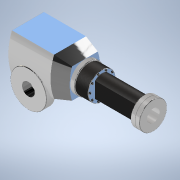
# Autodesk Inventor part: Part4
Saved by Autodesk Inventor 2022 (Build 260153000, 153)
## iProperties
Created: 2023-11-30
Part Number: Part4
Material: Generic
Document SubType Name: Modeling
Designer: harshidd
Density: 1 g/cm^3
Appearance: Aluminum - Polished
Author: harshidd
Autodesk Inventor part; units mm, degrees
sketch "Sketch1" plane through (0, 0, 0) normal (0, 0, 1) x (1, 0, 0)
  line L0 (0, 0) -> (0, 45) construction
  line L1 (0, 0) -> (0, -45) construction
  line L2 (0, 45) -> (37.5, 45)
  line L3 (37.5, 45) -> (-37.5, 45)
  line L4 (37.5, -45) -> (-37.5, -45)
  arc A0 (-37.5, 45) -> (-37.5, -45) centre (79.119038, 0) ccw
  arc A1 (37.5, -45) -> (37.5, 45) centre (-79.119038, 0) ccw
  dimension "d0" = 45
  dimension "d1" = 37.5
  dimension "d2" = 75
  dimension "d3" = 75
  dimension "d4" = 125
  dimension "d5" = 125
  constraints: 10 end point, 4 point on circle, 2 centre point, 2 vertical, 1 collinear, 1 horizontal, 1 point on line
  measures "d0" distance of L0.start L0.end
  measures "d1" distance of L0.end L2.end
  measures "d2" distance of L2.end L3.end
  measures "d3" distance of L4.start L4.end
  measures "d4" radius of A0
  measures "d5" radius of A1
sketch "Sketch1 outline for Extrusion1" plane through (0, 0, 0) normal (0, 0, 1) x (1, 0, 0)
  arc A0 (37.5, -45) -> (37.5, 45) centre (-79.119038, 0) ccw
  line L0 (-37.5, -45) -> (37.5, -45)
  arc A1 (-37.5, 45) -> (-37.5, -45) centre (79.119038, 0) ccw
  line L1 (37.5, 45) -> (-37.5, 45)
extrude "Extrusion1" add sketch "Sketch1 outline for Extrusion1" along normal blind 100
ref_plane "Work Plane1" through (0, 0, 135) normal (0, 0, 1) x (1, 0, 0)
sketch "Sketch2" plane through (0, 0, 135) normal (0, 0, 1) x (1, 0, 0)
  line L0 (37.5, 45) -> (-37.5, 45)
  arc A0 (-37.5, 45) -> (-37.5, -45) centre (79.119038, 0) ccw
  line L1 (-37.5, -45) -> (37.5, -45)
  arc A1 (37.5, -45) -> (37.5, 45) centre (-79.119038, 0) ccw
  line L2 (-30.425474, 35) -> (30.425474, 35)
  arc A2 (30.425474, -35) -> (30.425474, 35) centre (-79.119038, 0) ccw
  line L3 (30.425474, -35) -> (-30.425474, -35)
  arc A3 (-30.425474, 35) -> (-30.425474, -35) centre (79.119038, 0) ccw
  point P0 (0, 0)
  dimension "d9" = 10
  constraints: 4 end point, 4 point on circle, 2 centre point, 3 other
  measures "d9" distance between parallel lines of L0 L2
sketch "Sketch2 outline for Loft1" plane through (0, 0, 135) normal (0, 0, 1) x (1, 0, 0)
  line L0 (-30.425474, 35) -> (30.425474, 35)
  arc A0 (30.425474, 35) -> (30.425474, -35) centre (-79.119038, 0) cw
  line L1 (30.425474, -35) -> (-30.425474, -35)
  arc A1 (-30.425474, -35) -> (-30.425474, 35) centre (79.119038, 0) cw
loft "Loft1" add profiles "Sketch2 outline for Loft1" section 1 edges at (0, 45, 100) (-45.880962, 0, 100) (0, -45, 100) (45.880962, 0, 100)
sketch "Sketch3" plane through (-30.425474, 35, 135) normal (0, 0, 1) x (1, 0, 0)
  circle A0 centre (30.425474, -35) radius 34.5
  dimension "d14" = 69
  constraints: 1 centre point, 1 coincident
  measures "d14" diameter of A0
sketch "Sketch3 outline for Extrusion2" plane through (-30.425474, 35, 135) normal (0, 0, 1) x (1, 0, 0)
  circle A0 centre (30.425474, -35) radius 34.5
extrude "Extrusion2" add sketch "Sketch3 outline for Extrusion2" along normal blind 10
sketch "Sketch4" plane through (0, 0, 145) normal (0, 0, 1) x (1, 0, 0)
  circle A0 centre (0, 0) radius 34.5 projected
  circle A1 centre (0, 0) radius 32.5
  dimension "d17" = 2
  constraints: 1 centre point
  measures "d17" radial gap between concentric circles of A0 A1
sketch "Sketch4 outline for Extrusion3" plane through (0, 0, 145) normal (0, 0, 1) x (1, 0, 0)
  circle A0 centre (0, 0) radius 32.5
extrude "Extrusion3" add sketch "Sketch4 outline for Extrusion3" along normal blind 30
sketch "Sketch5" plane through (0, 0, 175) normal (0, 0, 1) x (1, 0, 0)
  line L0 (0, 0) -> (29, 0) construction
  circle A0 centre (29, 0) radius 2.5
  circle A1 centre (29, 0) radius 1.5
  dimension "d20" = 29
  dimension "d21" = 5
  dimension "d22" = 1
  constraints: 2 centre point, 2 end point, 1 coincident, 1 horizontal
  measures "d20" distance of L0.start L0.end
  measures "d21" diameter of A0
  measures "d22" radial gap between concentric circles of A0 A1
sketch "Sketch5 outline for Extrusion4" plane through (0, 0, 175) normal (0, 0, 1) x (1, 0, 0)
  circle A0 centre (29, 0) radius 2.5
  circle A1 centre (29, 0) radius 1.5
extrude "Extrusion4" add sketch "Sketch5 outline for Extrusion4" along normal blind 2
pattern_circular "Circular Pattern1" count 10 over 360 about axis through (0, 0, 145) along (0, 0, 1) of "Extrusion4"
sketch "Sketch6" plane through (0, 0, 175) normal (0, 0, 1) x (1, 0, 0)
  line L0 (0, 0) -> (16, 0) construction
  line L1 (16, 0) -> (16, 18.5) construction
  line L2 (16, 18.5) -> (16, -18.5)
  line L3 (0, 0) -> (0, -6.981731) construction
  line L4 (-16, 18.5) -> (-16, -18.5)
  arc A0 (16, 18.5) -> (-16, 18.5) centre (0, 4.898529) ccw
  arc A1 (-16, -18.5) -> (16, -18.5) centre (0, -4.898529) ccw
  dimension "d28" = 16
  dimension "d29" = 18.5
  dimension "d30" = 37
  dimension "d31" = 21
  dimension "d32" = 21
  constraints: 10 end point, 4 point on circle, 2 centre point, 2 symmetric about line, 2 vertical, 1 horizontal, 1 point on line
  measures "d28" distance of L0.start L0.end
  measures "d29" distance of L0.end L1.end
  measures "d30" distance of L1.end L2.end
  measures "d31" radius of A0
  measures "d32" radius of A1
sketch "Sketch6 outline for Extrusion5" plane through (0, 0, 175) normal (0, 0, 1) x (1, 0, 0)
  line L0 (16, 18.5) -> (16, -18.5)
  arc A0 (16, -18.5) -> (-16, -18.5) centre (0, -4.898529) cw
  line L1 (-16, -18.5) -> (-16, 18.5)
  arc A1 (-16, 18.5) -> (16, 18.5) centre (0, 4.898529) cw
extrude "Extrusion5" add sketch "Sketch6 outline for Extrusion5" along normal blind 100
sketch "Sketch7" plane through (0, 0, 275) normal (0, 0, 1) x (1, 0, 0)
  circle A0 centre (0, 0) radius 32.5 projected
sketch "Sketch7 outline for Extrusion6" plane through (0, 0, 275) normal (0, 0, 1) x (1, 0, 0)
  circle A0 centre (0, 0) radius 32.5
extrude "Extrusion6" add sketch "Sketch7 outline for Extrusion6" along normal blind 10
sketch "Sketch8" plane through (0, 0, 285) normal (0, 0, 1) x (1, 0, 0)
  circle A0 centre (0, 0) radius 32.5 projected
  circle A1 centre (0, 0) radius 31.5
  dimension "d37" = 1
  constraints: 1 centre point
  measures "d37" radial gap between concentric circles of A0 A1
sketch "Sketch8 outline for Extrusion7" plane through (0, 0, 285) normal (0, 0, 1) x (1, 0, 0)
  circle A0 centre (0, 0) radius 31.5
extrude "Extrusion7" add sketch "Sketch8 outline for Extrusion7" along normal blind 1
sketch "Sketch9" plane through (0, 0, 286) normal (0, 0, 1) x (1, 0, 0)
  circle A0 centre (0, 0) radius 32.5 projected
sketch "Sketch9 outline for Extrusion8" plane through (0, 0, 286) normal (0, 0, 1) x (1, 0, 0)
  circle A0 centre (0, 0) radius 32.5
extrude "Extrusion8" add sketch "Sketch9 outline for Extrusion8" along normal blind 10
ref_plane "Work Plane2" through (-37.5, -45, 50) normal (1, 0, 0) x (0, 1, 0)
sketch "Sketch10" plane through (-37.5, -45, 50) normal (1, 0, 0) x (0, 1, 0)
  line L0 (0, -50) -> (0, 50) projected
  circle A0 centre (0, 0) radius 42.5
  point P0 (45, -50)
  dimension "d42" = 85
  constraints: 1 centre point, 1 midpoint
  measures "d42" diameter of A0
sketch "Sketch10 outline for Extrusion9" plane through (-37.5, -45, 50) normal (1, 0, 0) x (0, 1, 0)
  circle A0 centre (0, 0) radius 42.5
extrude "Extrusion9" add sketch "Sketch10 outline for Extrusion9" along normal mid plane 21
sketch "Sketch11" plane through (-27, -45, 50) normal (1, 0, 0) x (0, 0, -1)
  line L0 (50, 0) -> (-50, 0) construction
  line L1 (0, 0) -> (0, -30) construction
  line L2 (20, 0) -> (20, -30)
  line L3 (-20, 0) -> (-20, -30)
  arc A0 (-20, -30) -> (20, -30) centre (0, -7.63932) ccw
  line L4 (-20, 0) -> (20, 0)
  point P0 (50, 45)
  dimension "d45" = 30
  dimension "d46" = 20
  dimension "d47" = 30
  constraints: 8 end point, 2 point on circle, 2 symmetric about line, 1 centre point, 1 collinear, 1 midpoint, 1 parallel, 1 vertical
  measures "d45" distance of L1.start L1.end
  measures "d46" distance between parallel lines of L1 L2
  measures "d47" radius of A0
sketch "Sketch11 outline for Extrusion10" plane through (-27, -45, 50) normal (1, 0, 0) x (0, 0, -1)
  line L0 (20, 0) -> (20, -30)
  arc A0 (20, -30) -> (-20, -30) centre (0, -7.63932) cw
  line L1 (-20, -30) -> (-20, 0)
  line L2 (-20, 0) -> (20, 0)
extrude "Extrusion10" add sketch "Sketch11 outline for Extrusion10" along normal blind 35
ref_plane "Work Plane3" through (8, -45, 50) normal (0, 0, 1) x (1, 0, 0)
sketch "Sketch12" plane through (8, -45, 50) normal (0, 0, 1) x (1, 0, 0)
  line L0 (0, -30) -> (0, 0)
  line L1 (0, 0) -> (0, -42)
  line L2 (0, 0) -> (25, 0)
  line L3 (-45.5, 0) -> (29.5, 0)
  arc A0 (0, -42) -> (25, 0) centre (-29.839254, 4.201937) ccw
  point P0 (-8, 45)
  dimension "d50" = 42
  dimension "d51" = 25
  dimension "d52" = 55
  constraints: 4 end point, 2 point on circle, 1 centre point, 1 collinear, 1 point on line
  measures "d50" distance of L0.end L1.end
  measures "d51" distance of L0.end L2.end
  measures "d52" radius of A0
sketch "Sketch12 outline for Extrusion11" plane through (8, -45, 50) normal (0, 0, 1) x (1, 0, 0)
  line L0 (25, 0) -> (0, 0)
  arc A0 (0, -42) -> (25, 0) centre (-29.839254, 4.201937) ccw
  line L1 (0, 0) -> (0, -42)
extrude "Extrusion11" add sketch "Sketch12 outline for Extrusion11" along normal mid plane 40
sketch "Sketch13" plane through (8, -87, 30) normal (-1, 0, 0) x (0, 0, 1)
  arc A0 (0, 12) -> (40, 12) centre (20, 34.36068) ccw
  line L0 (0, 0) -> (0, 12)
  line L1 (0, 0) -> (40, 0)
  line L2 (40, 12) -> (40, 0)
  point P0 (-30, 87)
sketch "Sketch13 outline for Extrusion12" plane through (8, -87, 30) normal (-1, 0, 0) x (0, 0, 1)
  line L0 (40, 0) -> (40, 12)
  line L1 (0, 0) -> (40, 0)
  line L2 (0, 12) -> (0, 0)
  arc A0 (40, 12) -> (0, 12) centre (20, 34.36068) cw
extrude "Extrusion12" cut sketch "Sketch13 outline for Extrusion12" against normal blind 40
fillet "Fillet1" radius 1 4 edges at (0, 45, 0) (45.881, 0, 0) (0, -45, 0) (-45.881, 0, 0)
fillet "Fillet2" radius 1 6 edges at (-48, -87.5, 50) (-27, -87.5, 50) (-34.5, 0, 145) (-32.5, 0, 175) (-32.5, 0, 296) (-32.5, 0, 275)
sketch "Sketch14" plane through (0, 0, 296) normal (0, 0, 1) x (1, 0, 0)
  circle A0 centre (0, 0) radius 15
  dimension "d59" = 30
  constraints: 1 centre point, 1 coincident
  measures "d59" diameter of A0
sketch "Sketch14 outline for Extrusion13" plane through (0, 0, 296) normal (0, 0, 1) x (1, 0, 0)
  circle A0 centre (0, 0) radius 15
extrude "Extrusion13" cut sketch "Sketch14 outline for Extrusion13" against normal blind 20
sketch "Sketch15" plane through (-48, -45, 50) normal (-1, 0, 0) x (0, 0, 1)
  line L0 (20, 0) -> (-20, 0) projected
  circle A0 centre (0, 0) radius 15
  point P0 (-50, 45)
  dimension "d62" = 30
  constraints: 1 centre point, 1 midpoint
  measures "d62" diameter of A0
sketch "Sketch15 outline for Extrusion14" plane through (-48, -45, 50) normal (-1, 0, 0) x (0, 0, 1)
  circle A0 centre (0, 0) radius 15
extrude "Extrusion14" cut sketch "Sketch15 outline for Extrusion14" against normal blind 20
body "Solid1"
